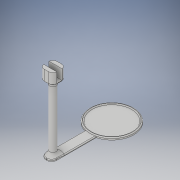
# Autodesk Inventor part: base2
Saved by Autodesk Inventor 2019 (Build 230136000, 136)
## iProperties
Created: 2020-10-30
Part Number: base2
Material: Generic
Document SubType Name: Modeling
Designer: Mike
Density: 1 g/cm^3
Appearance: Default
Author: Mike
## iProperties of the stored document base2_3DPrint.ipt
Created: 2020-11-05
Part Number: base2_3DPrint
Material: Generic
Document SubType Name: Modeling
Designer: Mike
Density: 1 g/cm^3
Appearance: Default
Author: Mike
Autodesk Inventor part; units mm, degrees
ref_plane "YZ Plane" through (0, 0, 0) normal (1, 0, 0) x (0, 1, 0)
ref_plane "XZ Plane" through (0, 0, 0) normal (0, 1, 0) x (-1, 0, 0)
ref_plane "XY Plane" through (0, 0, 0) normal (0, 0, 1) x (1, 0, 0)
sketch "Sketch1" plane through (0, 0, 0) normal (0, 1, 0) x (-1, 0, 0)
  line L0 (0, 0) -> (-25, 0)
  line L1 (-25, 0) -> (-25, -150)
  line L2 (-25, -150) -> (0, -150)
  line L3 (0, -150) -> (0, 0)
  dimension "d0" = 25
  dimension "d1" = 150
  constraints: 8 end point, 2 parallel, 1 horizontal, 1 perpendicular
  measures "d0" distance of L2.end L1.end
  measures "d1" distance of L1.end L0.end
extrude "Extrusion1" add sketch "Sketch1" along normal blind 3
sketch "Sketch2" plane through (0, 3, 0) normal (0, 1, 0) x (1, 0, 0)
  line L0 (0, 0) -> (25, 0) projected
  line L1 (25, 0) -> (25, 150) projected
  line L2 (25, 150) -> (0, 150) projected
  line L3 (0, 150) -> (0, 0) projected
  line L4 (12.5, 0) -> (12.5, 15)
  circle A0 centre (12.5, 15) radius 7.5
  dimension "d4" = 15
  dimension "d5" = 15
  constraints: 2 end point, 1 centre point, 1 coincident, 1 midpoint, 1 perpendicular
  measures "d4" distance of L4.start L4.end
  measures "d5" diameter of A0
extrude "Extrusion2" add sketch "Sketch2" along normal blind 150 contours A0
sketch "Sketch3" plane through (12.5, 153, -15) normal (0, 1, 0) x (1, 0, 0)
  line L0 (-15, -15) -> (15, -15)
  line L1 (15, -15) -> (15, 15)
  line L2 (15, 15) -> (-15, 15)
  line L3 (-15, 15) -> (-15, -15)
  circle A0 centre (0, 0) radius 7.5 projected
  line L4 (-12.5, -15) -> (12.5, -15) projected
  dimension "d8" = 30
  dimension "d9" = 30
  dimension "d10" = 15
  dimension "d11" = 0
  constraints: 8 end point, 2 parallel, 1 horizontal, 1 perpendicular
  measures "d8" distance of L2.end L1.end
  measures "d9" distance of L1.end L0.end
  measures "d10" distance from line of L3 A0.centre
  measures "d11" distance between parallel lines of L4 L0
extrude "Extrusion3" add sketch "Sketch3" along normal blind 2 contours L3 L2 L1 L0 | A0
sketch "Sketch4" plane through (12.5, 155, -15) normal (0, 1, 0) x (1, 0, 0)
  line L0 (-15, -15) -> (15, -15) projected
  line L1 (15, -15) -> (15, 15) projected
  line L2 (15, 15) -> (-15, 15) projected
  line L3 (-15, 15) -> (-15, -15) projected
  line L4 (-15, -6.1) -> (15, -6.1)
  line L5 (15, -6.1) -> (15, 6.1)
  line L6 (15, 6.1) -> (-15, 6.1)
  line L7 (-15, 6.1) -> (-15, -6.1)
  point P0 (-12.5, -15)
  dimension "d14" = 12.2
  dimension "d15" = 0
  dimension "d16" = 0
  dimension "d17" = 30
  dimension "d18" = 8.9
  constraints: 8 end point, 2 parallel, 1 horizontal, 1 perpendicular
  measures "d14" distance of L4.end L5.end
  measures "d15" distance between parallel lines of L3 L7
  measures "d16" distance between parallel lines of L5 L1
  measures "d17" distance between parallel lines of L2 L0
  measures "d18" distance between parallel lines of L4 L0
extrude "Extrusion4" add sketch "Sketch4" along normal blind 23 contours L3 L4 L1 L0 | L3 L2 L1 L6
fillet "Fillet1" radius 10 1 edges at (5, 3, -15)
fillet "Fillet2" radius 10 1 edges at (5, 153, -15)
fillet "Fillet3" radius 10 4 edges at (27.5, 165.5, 0) (-2.5, 165.5, 0) (27.5, 165.5, -30) (-2.5, 165.5, -30)
fillet "Fillet4" [suppressed]
fillet "Fillet5" radius 12 2 edges at (25, 1.5, 0) (0, 1.5, 0)
sketch "Sketch5" plane through (0, 3, 0) normal (0, 1, 0) x (1, 0, 0)
  line L0 (25, 150) -> (0, 150) projected
  circle A0 centre (12.5, 150) radius 50
  point P0 (0, 0)
  dimension "d26" = 100
  constraints: 1 centre point, 1 midpoint
  measures "d26" diameter of A0
extrude "Extrusion5" add sketch "Sketch5" against normal up to surface (3 mm away)
sketch "Sketch6" plane through (0, 3, 0) normal (0, 1, 0) x (1, 0, 0)
  arc A0 (25, 101.5877) -> (0, 101.5877) centre (12.5, 150) ccw projected
  circle A1 centre (12.5, 150) radius 50
  circle A2 centre (12.5, 150) radius 45
  point P0 (0, 0)
  dimension "d29" = 5
  constraints: 2 centre point, 2 coincident, 1 concentric
  measures "d29" radial gap between concentric circles of A1 A2
extrude "Extrusion6" add sketch "Sketch6" along normal blind 2
fillet "Fillet6" radius 2 2 edges at (-37.5, 5, -150) (-32.5, 5, -150)
fillet "Fillet8" radius 2 9 edges at (27.5, 152.7336, -12.4988) (27.5, 152.7336, -17.5012) (24.5711, 152.9908, -27.0711) (12.5, 152.6825, -30) (0.4289, 152.9908, -27.0711) (-2.5, 152.6825, -15) (0.4289, 152.9908, -2.9289) (12.5, 152.6825, 0) (24.5711, 152.9908, -2.9289)
fillet "Fillet9" radius 2 8 edges at (12.5, 3.3175, 0) (3.4935, 3.4362, -3.536) (0, 3.9095, -19.6393) (0, 3, -64.4176) (25, 3.6631, -21.123) (25, 4.2884, -13.497) (25, 3, -64.4176) (21.5064, 3.4362, -3.5358)
equation "\"d9\" = d8"
equation "\"d10\" = 0.5 * d8"
equation "\"d18\" = -0.5 * d14 + 0.5 * d17"
body "Solid1"
